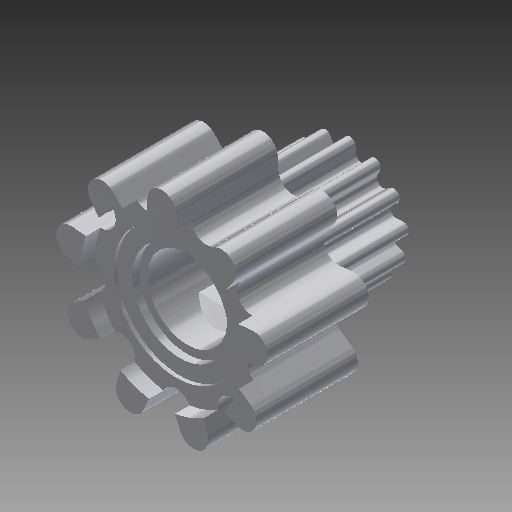
# Autodesk Inventor part: 402-05
Saved by Autodesk Inventor 2019 (Build 230136000, 136)
## iProperties
Company: Autodesk Inc.
Created: 2017-06-27
Part Number: 402-05
Material: PVC-U
Document SubType Name: Modeling
Designer: Autodesk Inc.
Mass: 1.04226 g
Surface Area: 10.7861 cm^2
Volume: 0.807952 cm^3
Density: 1.29 g/cm^3
Appearance: Smooth - White
Author: Inventor
Autodesk Inventor part; units mm, degrees
ref_plane "YZ Plane" through (0, 0, 0) normal (1, 0, 0) x (0, 1, 0)
ref_plane "XZ Plane" through (0, 0, 0) normal (0, 1, 0) x (-1, 0, 0)
ref_plane "XY Plane" through (0, 0, 0) normal (0, 0, 1) x (1, 0, 0)
sketch "Sketch1" plane through (0, 0, 0) normal (0, 0, 1) x (1, 0, 0)
  line L0 (0, 0) -> (-1.7101, 4.6985)
  line L1 (0, 0) -> (1.7101, 4.6985)
  line L2 (0, 0) -> (0, 6.4) construction
  circle A0 centre (0, 6.4) radius 1
  circle A1 centre (-2.0521, 5.6382) radius 1
  circle A2 centre (2.0521, 5.6382) radius 1
  line L3 (-2.0521, 5.6382) -> (2.0521, 5.6382) construction
  circle A3 centre (0, 0) radius 5 construction
  circle A4 centre (0, 0) radius 7.4 construction
  line L4 (-1.0541, 5.5751) -> (-0.998, 6.4631)
  line L5 (1.0541, 5.5751) -> (0.998, 6.4631)
  line L6 (-1.7101, 4.6985) -> (-2.0521, 5.6382) construction
  line L7 (1.7101, 4.6985) -> (2.0521, 5.6382) construction
  point P0 (0, 5.6382)
  dimension "d0" = 2
  dimension "d1" = 40
  dimension "d2" = 10
  dimension "d3" = 14.8
  constraints: 16 end point, 6 point on circle, 6 tangent, 5 centre point, 4 coincident, 2 collinear, 2 equal radius, 1 midpoint, 1 perpendicular, 1 point on line, 1 vertical
  measures "d0" diameter of A0
  measures "d1" angle of L0 L1
  measures "d2" diameter of A3
  measures "d3" diameter of A4
extrude "Extrusion1" add sketch "Sketch1" along normal blind 7 contours L0 A1 L4 A0 L5 A2 L1 | A0
pattern_circular "Circular Pattern1" count 9 over 360 about axis through (0, 0, 0) along (0, 0, 1)
sketch "Sketch2" plane through (0, 0, 0) normal (0, 0, 1) x (1, 0, 0)
  circle A0 centre (0, 0) radius 4.1 construction
  circle A1 centre (0, 0) radius 3 construction
  line L0 (0, 0) -> (0, 3.7) construction
  line L1 (0.7179, 2.9128) -> (0.8137, 3.3012) construction
  line L2 (-0.7179, 2.9128) -> (-0.8137, 3.3012) construction
  line L3 (-0.8137, 3.3012) -> (-0.7179, 2.9128) construction
  line L4 (0, 0) -> (0.7179, 2.9128)
  circle A2 centre (0, 3.7) radius 0.4
  arc A3 (0.4139, 3.2879) -> (0.7179, 2.9128) centre (0.8137, 3.3012) ccw
  arc A4 (-0.7179, 2.9128) -> (-0.4139, 3.2879) centre (-0.8137, 3.3012) ccw
  line L5 (0.4139, 3.2879) -> (0.3998, 3.7133)
  line L6 (-0.4139, 3.2879) -> (-0.3998, 3.7133)
  line L7 (0, 0) -> (-0.7179, 2.9128)
  dimension "d9" = 8.2
  dimension "d10" = 6
  dimension "d11" = 0.8
  dimension "d13" = 27.692
  constraints: 16 end point, 8 point on circle, 7 tangent, 5 centre point, 5 coincident, 3 collinear, 2 equal radius, 2 point on line, 1 horizontal alignment, 1 vertical
  measures "d9" diameter of A0
  measures "d10" diameter of A1
  measures "d11" diameter of A2
  measures "d13" angle of L1 L2
extrude "Extrusion2" add sketch "Sketch2" against normal blind 6
pattern_circular "Circular Pattern2" count 13 over 360 about axis through (0, 0, 0) along (0, 0, -1) of "Extrusion2"
sketch "Sketch3" plane through (0, 0, 0) normal (1, 0, 0) x (0, 1, 0)
  line L0 (0, 0) -> (1.5, 0)
  line L1 (1.5, 0) -> (1.5, -6)
  line L2 (1.5, -6) -> (0, -6)
  line L3 (0, -6) -> (0, 0)
  line L4 (0, 0) -> (2.75, 0)
  line L5 (2.75, 0) -> (2.75, 5.25)
  line L6 (2.75, 5.25) -> (0, 5.25)
  line L7 (0, 5.25) -> (0, 0)
  line L8 (0, 5.25) -> (3.3, 5.25)
  line L9 (3.3, 5.25) -> (3.3, 5.75)
  line L10 (3.3, 5.75) -> (0, 5.75)
  line L11 (0, 5.75) -> (0, 5.25)
  line L12 (0, 5.75) -> (4.35, 5.75)
  line L13 (4.35, 5.75) -> (4.35, 6)
  line L14 (4.35, 6) -> (0, 6)
  line L15 (0, 6) -> (0, 5.75)
  line L16 (0, 6) -> (5.625, 6)
  line L17 (5.625, 6) -> (5.625, 7)
  line L18 (5.625, 7) -> (0, 7)
  line L19 (0, 7) -> (0, 6)
  dimension "d19" = 7
  dimension "d20" = 6
  dimension "d22" = 11.25
  dimension "d23" = 1
  dimension "d24" = 8.7
  dimension "d25" = 1.25
  dimension "d27" = 6.6
  dimension "d28" = 3
  dimension "d29" = 5.5
  dimension "d30" = 1.75
  constraints: 40 end point, 10 parallel, 5 horizontal, 5 perpendicular
  measures "d19" distance from line of L18 L0.start
  measures "d20" distance of L2.end L0.start
  measures "d22" diameter of L17 L19
  measures "d23" distance of L16.end L17.end
  measures "d24" diameter of L13 L19
  measures "d25" distance between parallel lines of L12 L18
  measures "d27" diameter of L9 L19
  measures "d28" diameter of L1 L3
  measures "d29" diameter of L5 L19
  measures "d30" distance between parallel lines of L8 L18
revolve "Revolution1" cut sketch "Sketch3" angle 360 about axis through (0, 0, 5.25) along (0, 0, -1)
sketch "Sketch4" plane through (0, 0, 0) normal (1, 0, 0) x (0, 1, 0)
  line L0 (2.75, 0) -> (-2.75, 0) projected
  line L1 (2.75, 0) -> (2.75, 5.25) projected
  line L2 (-2.75, 0) -> (-2.75, 5.25) projected
  line L3 (1.95, 0) -> (1.95, 2.5)
  line L4 (-1.95, 0) -> (-1.95, 2.5)
  line L5 (-1.95, 2.5) -> (-2.75, 3.3)
  line L6 (1.95, 2.5) -> (2.75, 3.3)
  point P0 (0, 0)
  dimension "d32" = 3.9
  dimension "d33" = 2.5
  dimension "d34" = 45
  constraints: 8 end point, 4 point on line, 2 horizontal alignment, 2 parallel, 1 perpendicular
  measures "d32" distance between parallel lines of L3 L4
  measures "d33" distance of L4.start L4.end
  measures "d34" angle of L5 L4
extrude "Extrusion3" add sketch "Sketch4" along normal through all both and the other way through all
body "Solid1"
